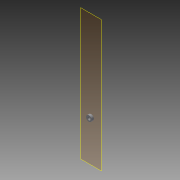
# Autodesk Inventor part: short spacer
Saved by Autodesk Inventor 2015 (Build 190159000, 159)
## iProperties
Created: 2014-11-22
Part Number: short spacer
Material: Generic
Document SubType Name: Modeling
Designer: jesse
Density: 1 g/cm^3
Appearance: Default
Author: jesse
Autodesk Inventor part; units mm, degrees
ref_plane "YZ Plane" through (0, 0, 0) normal (1, 0, 0) x (0, 1, 0)
ref_plane "XZ Plane" through (0, 0, 0) normal (0, 1, 0) x (-1, 0, 0)
ref_plane "Work Plane1" through (0, 0, -289.9906) normal (0, 0, 1) x (1, 0, 0)
sketch "Sketch1" plane through (0, 0, -289.9906) normal (0, 0, 1) x (1, 0, 0)
  circle A0 centre (12.7, 70.6437) radius 3.175 projected
  circle A1 centre (12.7, 167.1637) radius 3.175 projected
  line L0 (25.4, 0) -> (0, 0) projected
  line L1 (25.4, 0) -> (25.4, 237.8075) projected
  line L2 (0, 237.8075) -> (25.4, 237.8075) projected
  line L3 (0, 0) -> (0, 237.8075) projected
  circle A2 centre (12.7, 70.6437) radius 5.6544
  constraints: 1 centre point, 1 coincident
ref_plane "Work Plane2" through (-6.2061, 45.3877, 4.4506) normal (0, 0, -1) x (0.3131, 0.9497, 0)
extrude "Extrusion1" add sketch "Sketch1" along normal up to surface (294.4412 mm away) contours A2
body "Solid1"
